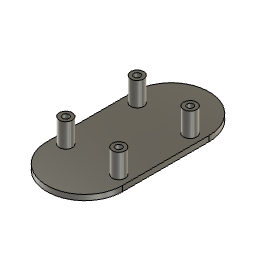
Wheel_mount (Autodesk Fusion 360 design; units mm, degrees)
Autodesk Fusion 360 part; units mm, degrees
sketch "Sketch1" plane through (0, 0, 0) normal (0, 0, 1) x (1, 0, 0)
  line L0 (35, 40) -> (35, -40)
  line L1 (-35, -40) -> (-35, 40)
  line L2 (0, 1.75) -> (0, 22.5)
  line L3 (1.75, 0) -> (22.5, 0)
  arc A0 (-35, -40) -> (35, -40) centre (0, -40) ccw
  arc A1 (35, 40) -> (-35, 40) centre (0, 40) ccw
  dimension "d2" = 80
  dimension "d3" = 70
  constraint vertical L0
  constraint vertical L1
  constraint symmetric L0 L1 L2
  constraint tangent L1 A1
  constraint tangent L0 A1
  constraint tangent L0 A0
  constraint tangent L1 A0
  constraint symmetric L3 A0 A1
  measures "d2" distance of L0.start L0.end
  measures "d3" distance of L0 L1
extrude "Extrude1" add sketch "Sketch1" along normal blind 5
sketch "Sketch2" plane through (0, 0, 5) normal (0, 0, 1) x (-1, 0, 0)
  arc A0 (35, 40) -> (-35, 40) centre (0, 40) ccw
  line L0 (-35, 40) -> (-35, -40)
  arc A1 (-35, -40) -> (35, -40) centre (0, -40) ccw
  line L1 (35, -40) -> (35, 40)
  line L2 (24.5, -33) -> (-24.5, -33) construction
  line L3 (-24.5, -33) -> (-24.5, 33) construction
  line L4 (-24.5, 33) -> (24.5, 33) construction
  line L5 (24.5, 33) -> (24.5, -33) construction
  line L6 (-1.75, 0) -> (-22.5, 0)
  line L7 (0, -1.75) -> (0, -22.5)
  point P0 (24.5, -33)
  point P1 (-24.5, -33)
  point P2 (-24.5, 33)
  point P3 (24.5, 33)
  dimension "d6" = 49
  dimension "d7" = 66
  constraint horizontal L2
  constraint vertical L3
  constraint horizontal L4
  constraint vertical L5
  constraint coincident P0 L2.start
  constraint coincident P1 L2.end
  constraint coincident P2 L3.end
  constraint coincident P3 L4.end
  constraint symmetric L2 L4 L6
  constraint symmetric L3 L5 L7
  measures "d6" distance of P0 P1
  measures "d7" distance of P0 P3
hole "Hole1" at (-24.5, 33, 5) at (24.5, 33, 5) at (24.5, -33, 5) at (-24.5, -33, 5) direction (0, 0, -1) diameter 6 end through all
sketch "Sketch3" plane through (0, 0, 5) normal (0, 0, 1) x (-1, 0, 0)
  circle A0 centre (-24.5, 33) radius 3
  circle A1 centre (24.5, -33) radius 3
  circle A2 centre (-24.5, -33) radius 3
  circle A3 centre (24.5, 33) radius 3
  arc A4 (35, 40) -> (-35, 40) centre (0, 40) ccw
  line L0 (-35, 40) -> (-35, -40)
  arc A5 (-35, -40) -> (35, -40) centre (0, -40) ccw
  line L1 (35, -40) -> (35, 40)
  circle A6 centre (24.5, -33) radius 3
  circle A7 centre (-24.5, -33) radius 3
  circle A8 centre (-24.5, 33) radius 3
  circle A9 centre (24.5, 33) radius 3
  circle A10 centre (24.5, -33) radius 6
  circle A11 centre (-24.5, -33) radius 6
  circle A12 centre (24.5, 33) radius 6
  circle A13 centre (-24.5, 33) radius 6
  dimension "d10" = 3
  dimension "d11" = 3
  dimension "d12" = 3
  dimension "d13" = 3
  measures "d10" distance of A1
  measures "d11" distance of A2
  measures "d12" distance of A3
  measures "d13" distance of A0
extrude "Extrude2" add sketch "Sketch3" along normal blind 22 contours A10 | A11 | A12 | A13
